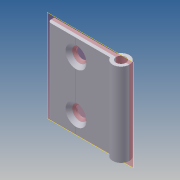
# Autodesk Inventor part: 23-225Z1
Saved by Autodesk Inventor 2011 SP2 (Build 150309200, 309)
## iProperties
Created: 2011-01-12
Part Number: 23-225Z1
Material: Aluminum-6061
Document SubType Name: Modeling
Designer: dc85560
Stock Number: 23-225Z1
Mass: 25.4335 g
Surface Area: 65.8844 cm^2
Volume: 9.38507 cm^3
Density: 2.71 g/cm^3
Title: Concealed Hinge 40, Half Hinge
Author: dc85560
Autodesk Inventor part; units mm, degrees
ref_plane "XZ Plane" through (0, 0, 0) normal (0, 1, 0) x (-1, 0, 0)
sketch "Sketch1" plane through (0, 0, 0) normal (0, 0, 1) x (1, 0, 0)
  circle A0 centre (0, 0) radius 5
  dimension "d0" = 10
  constraints: 1 centre point, 1 coincident
  measures "d0" diameter of A0
extrude "Extrusion1" add sketch "Sketch1" against normal blind 50
ref_plane "Work Plane1" through (-42, 0, 0) normal (1, 0, 0) x (0, 1, 0)
sketch "Sketch2" plane through (-42, 0, 0) normal (1, 0, 0) x (0, 1, 0)
  line L0 (5, -50) -> (-5, -50) projected
  line L1 (-5, 0) -> (5, 0) projected
  line L2 (0, -60) -> (0, 10) projected
  line L3 (-2, 0) -> (2, 0)
  line L4 (2, 0) -> (2, -50)
  line L5 (2, -50) -> (-2, -50)
  line L6 (-2, -50) -> (-2, 0)
  dimension "d4" = 4
  dimension "d5" = 2
  constraints: 8 end point, 2 parallel, 2 point on line, 1 horizontal, 1 perpendicular
  measures "d4" distance of L3.start L3.end
  measures "d5" distance between parallel lines of L2 L6
extrude "Extrusion2" add sketch "Sketch2" along normal blind 42
sketch "Sketch3" plane through (0, 0, 0) normal (0, 0, 1) x (1, 0, 0)
  arc A0 (-4.5826, -2) -> (-4.5826, 2) centre (0, 0) ccw projected
hole "Hole1" at (0, 0, 0) direction (0, 0, -1) diameter 6 end through all
ref_plane "Work Plane2" through (-25, 0, 0) normal (1, 0, 0) x (0, 1, 0)
sketch "Sketch4" plane through (-42, -2, -50) normal (0, -1, 0) x (1, 0, 0)
  line L0 (0, 0) -> (37.4174, 0) projected
  line L1 (17, 60) -> (17, -10) projected
  point P0 (17, 40)
  point P1 (17, 10)
  dimension "d16" = 30
  dimension "d17" = 10
  constraints: 2 point on line
  measures "d16" distance of point (17, 10) point (17, 40)
  measures "d17" distance from line of L0 point (17, 10)
hole "Hole2" at (-25, -2, -10) at (-25, -2, -40) direction (0, 1, 0) diameter 6.4 end through all countersink diameter 12.6 countersink angle 90 clearance for "Flat Head Machine Screw" size "M6" standard "Ansi Metric M Profile"
sketch "Sketch5" plane through (0, 0, -50) normal (0, 0, -1) x (-1, 0, 0)
  line L0 (42, -2) -> (4.5826, -2) projected
  line L1 (25, -7) -> (25, 7) projected
  line L2 (24.9, -2) -> (25, -1.9)
  line L3 (25, -1.9) -> (25.1, -2)
  dimension "d25" = 90
  dimension "d26" = 45
  dimension "d27" = 0.1
  constraints: 4 end point, 3 point on line
  measures "d25" angle of L3 L2
  measures "d26" angle of L1 L2
  measures "d27" distance from line of L2.end L0
extrude "Extrusion3" cut sketch "Sketch5" against normal through all
fillet "Fillet1" radius 2 1 edges at (-42, -2, -25)
equation "\"d5\" = 0.5 * d4"
equation "\"d26\" = 0.5 * d25"
body "Solid1"
